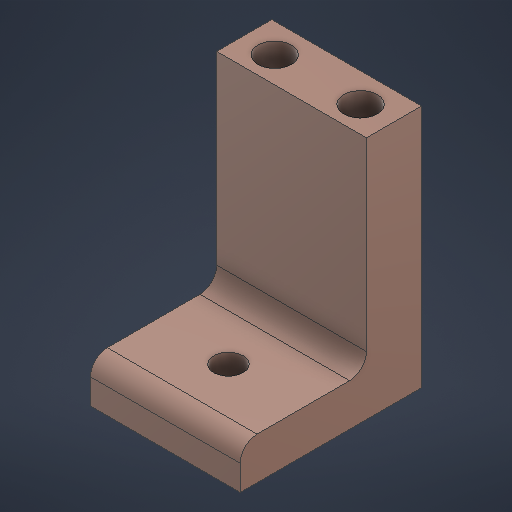
# Autodesk Inventor part: Sujeción de servo a mesa s-c
Saved by Autodesk Inventor 2026 (Build 300175000, 175)
## iProperties
Created: 2025-08-24
Part Number: Sujeción de servo a mesa s-c
Material: Plástico PC/ABS
Document SubType Name: Modeling
Designer: Thomas
Density: 1.1 g/cm^3
Appearance: Suave - Blanco
Author: Thomas
Autodesk Inventor part; units mm, degrees
ref_plane "YZ Plane" through (0, 0, 0) normal (1, 0, 0) x (0, 1, 0)
ref_plane "XZ Plane" through (0, 0, 0) normal (0, 1, 0) x (-1, 0, 0)
ref_plane "XY Plane" through (0, 0, 0) normal (0, 0, 1) x (1, 0, 0)
sketch "Boceto1" plane through (0, 0, 0) normal (1, 0, 0) x (0, 1, 0)
  line L0 (27, 0) -> (0, 0)
  line L1 (0, 0) -> (0, 6.55)
  line L2 (0, 6.55) -> (27, 6.55)
  line L3 (27, 6.55) -> (27, 0)
  line L4 (0, 6.55) -> (5, 6.55)
  line L5 (5, 6.55) -> (5, 21.55)
  line L6 (5, 21.55) -> (0, 21.55)
  line L7 (0, 21.55) -> (0, 6.55)
  dimension "d0" = 27
  dimension "d1" = 6.55
  dimension "d2" = 15
  dimension "d3" = 5
  constraints: 16 end point, 4 parallel, 2 horizontal, 2 perpendicular, 1 coincident
  measures "d0" distance of L0.start L0.end
  measures "d1" distance of L2.end L0.start
  measures "d2" distance of L4.end L5.end
  measures "d3" distance of L5.end L6.end
extrude "Extrusión1" add sketch "Boceto1" along normal mid plane 17.8
sketch "Boceto4" plane through (-8.9, 5, 21.55) normal (0, 1, 0) x (1, 0, 0)
  point P0 (8.9, 21.55)
sketch "Boceto5" plane through (-8.9, 27, 6.55) normal (0, 1, 0) x (1, 0, 0)
  circle A0 centre (3.8, 3.1) radius 2
  circle A1 centre (14, 3.1) radius 2
  line L0 (0, 0) -> (17.8, 0) projected
  line L1 (0, 0) -> (0, 6.55) projected
  line L2 (17.8, 6.55) -> (17.8, 0) projected
  point P0 (8.9, 6.55)
  dimension "d10" = 4
  dimension "d11" = 4
  dimension "d12" = 3.1
  dimension "d13" = 3.8
  dimension "d14" = 3.8
  constraints: 2 centre point, 1 horizontal alignment
  measures "d10" diameter of A0
  measures "d11" diameter of A1
  measures "d12" distance from line of A0.centre L0
  measures "d13" distance from line of A0.centre L1
  measures "d14" distance from line of A1.centre L2
extrude "Extrusión3" cut sketch "Boceto5" against normal blind 10
sketch "Boceto6" plane through (-8.9, 5, 21.55) normal (0, 1, 0) x (1, 0, 0)
  circle A0 centre (8.9, 7.5) radius 1.75
  line L0 (0, 0) -> (0, 15) projected
  line L1 (0, 0) -> (17.8, 0) projected
  point P0 (8.9, 21.55)
  point P1 (0, 7.5)
  point P2 (8.9, 0)
  dimension "d17" = 3.5
  constraints: 2 midpoint, 1 centre point, 1 horizontal alignment, 1 vertical alignment
  measures "d17" diameter of A0
extrude "Extrusión4" cut sketch "Boceto6" against normal blind 10
fillet "Empalme1" radius 2 1 edges at (0, 5, 6.55)
fillet "Empalme2" radius 2 1 edges at (0, 5, 21.55)
move faces "Desplazar1" translate (0, 2, 0) faces at (1.6196, 27, 0.4882)
equation "\"d11\" = d10"
equation "\"d14\" = d13"
